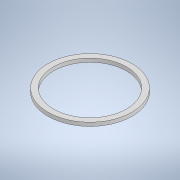
# Autodesk Inventor part: backup_ring
Saved by Autodesk Inventor 2020 (Build 240168000, 168)
## iProperties
Created: 2020-06-29
Part Number: backup_ring
Material: Generic
Document SubType Name: Modeling
Designer: minso
Density: 1 g/cm^3
Appearance: Default
Author: minso
Autodesk Inventor part; units mm, degrees
ref_plane "YZ Plane" through (0, 0, 0) normal (1, 0, 0) x (0, 1, 0)
ref_plane "XZ Plane" through (0, 0, 0) normal (0, 1, 0) x (-1, 0, 0)
ref_plane "XY Plane" through (0, 0, 0) normal (0, 0, 1) x (1, 0, 0)
sketch "Sketch1" plane through (0, 0, 0) normal (0, 0, 1) x (1, 0, 0)
  line L0 (100, 5) -> (115, 5)
  line L1 (115, 5) -> (115, -5)
  line L2 (115, -5) -> (100, -5)
  line L3 (100, -5) -> (100, 5)
  line L4 (0, 4.5532) -> (0, -4.5532)
  point P0 (0, 0)
  point P1 (0, 0)
  point P2 (100, 0)
  dimension "fascia_parameter" = 15
  dimension "height_parameter" = 10
  dimension "externalDiameter_parameter" = 230
  constraints: 10 end point, 2 coincident, 2 midpoint, 2 parallel, 1 horizontal, 1 horizontal alignment, 1 perpendicular, 1 vertical
  measures "fascia_parameter" distance of L0.start L0.end
  measures "height_parameter" distance of L0.end L1.end
  measures "externalDiameter_parameter" diameter of L1 L4
revolve "Revolution1" add sketch "Sketch1" angle 360 about axis through (0, 4.5532, 0) along (0, -1, 0)
body "Solid1"
